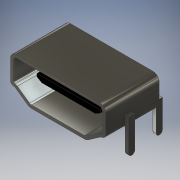
# Autodesk Inventor part: HDMI_Conn
Saved by Autodesk Inventor 2016 (Build 200138000, 138)
## iProperties
Created: 2017-03-02
Part Number: HDMI_Conn
Material: Generic
Document SubType Name: Modeling
Designer: jfixelle
Density: 1 g/cm^3
Appearance: Default
Author: jfixelle
Autodesk Inventor part; units mm, degrees
sketch "Sketch1" plane through (0, 0, 0) normal (0, 0, 1) x (1, 0, 0)
  line L0 (-6.5, 3.1) -> (6.5, 3.1)
  line L1 (7.5, 2.1) -> (7.5, -0.941077)
  line L2 (4.184701, -3.1) -> (-4.184701, -3.1)
  line L3 (-7.5, -0.941077) -> (-7.5, 2.1)
  line L4 (-4.758278, -2.919152) -> (-6.675075, -1.576996)
  line L5 (4.758278, -2.919152) -> (6.675075, -1.576996)
  line L6 (-6.747295, -1.526427) -> (-6.402425, -1.033902)
  line L7 (-6.747295, -1.526427) -> (6.747295, -1.526427)
  line L8 (6.832454, -1.503609) -> (7.12941, -1.42404)
  line L9 (-6.832454, -1.503609) -> (-7.12941, -1.42404)
  arc A0 (-6.675075, -1.576996) -> (-6.832454, -1.503609) centre (-6.961864, -1.986572) ccw
  arc A1 (-7.5, -0.941077) -> (-7.12941, -1.42404) centre (-7, -0.941077) ccw
  arc A2 (6.832454, -1.503609) -> (6.675075, -1.576996) centre (6.961864, -1.986572) ccw
  arc A3 (7.12941, -1.42404) -> (7.5, -0.941077) centre (7, -0.941077) ccw
  arc A4 (-6.5, 3.1) -> (-7.5, 2.1) centre (-6.5, 2.1) ccw
  arc A5 (7.5, 2.1) -> (6.5, 3.1) centre (6.5, 2.1) ccw
  arc A6 (4.184701, -3.1) -> (4.758278, -2.919152) centre (4.184701, -2.1) ccw
  arc A7 (-4.758278, -2.919152) -> (-4.184701, -3.1) centre (-4.184701, -2.1) ccw
  line L10 (-7, 2.1) -> (-7, -0.749246)
  arc A8 (-7, -0.941077) -> (-7, -0.941077) centre (-7, -0.941077) ccw
  line L11 (-6.814705, -0.990727) -> (-6.703044, -1.020646)
  arc A9 (-6.388287, -1.16742) -> (-6.703044, -1.020646) centre (-6.961864, -1.986572) ccw
  line L12 (-6.388287, -1.16742) -> (-4.471489, -2.509576)
  arc A10 (-4.471489, -2.509576) -> (-4.184701, -2.6) centre (-4.184701, -2.1) ccw
  line L13 (-4.184701, -2.6) -> (4.184701, -2.6)
  arc A11 (4.184701, -2.6) -> (4.471489, -2.509576) centre (4.184701, -2.1) ccw
  line L14 (4.471489, -2.509576) -> (6.388287, -1.16742)
  arc A12 (6.703044, -1.020646) -> (6.388287, -1.16742) centre (6.961864, -1.986572) ccw
  line L15 (6.703044, -1.020646) -> (6.814705, -0.990727)
  arc A13 (7, -0.941077) -> (7, -0.941077) centre (7, -0.941077) ccw
  line L16 (7, -0.749246) -> (7, 2.1)
  arc A14 (7, 2.1) -> (6.5, 2.6) centre (6.5, 2.1) ccw
  line L17 (6.5, 2.6) -> (-6.5, 2.6)
  arc A15 (-6.5, 2.6) -> (-7, 2.1) centre (-6.5, 2.1) ccw
  arc A16 (-7, -0.749246) -> (-6.814705, -0.990727) centre (-6.75, -0.749246) ccw
  arc A17 (6.814705, -0.990727) -> (7, -0.749246) centre (6.750001, -0.749246) ccw
  point P0 (0, 0)
  point P1 (-7.5, 3.1)
  point P2 (7.5, -3.1)
  point P3 (7.5, 3.1)
  point P4 (-7.5, -3.1)
  point P5 (-4.5, -3.1)
  point P6 (-7.5, -0.999377)
  point P7 (4.5, -3.1)
  point P8 (7.5, -0.999377)
  dimension "d1" = 15
  dimension "d2" = 7.5
  dimension "d3" = 6.2
  dimension "d4" = 3.1
  dimension "d5" = 9
  dimension "d6" = 4.5
  dimension "d7" = 35
  dimension "d8" = 35
  dimension "d11" = 90
  dimension "d12" = 0.52705
  dimension "d13" = 15
  dimension "d14" = 15
  dimension "d15" = 0.5
  dimension "d16" = 1
  dimension "d17" = 14
  dimension "d18" = 0.25
  constraints: 36 end point, 32 point on circle, 24 point on line, 20 tangent, 18 centre point, 7 equal radius, 4 coincident with centre, 4 parallel, 3 perpendicular, 1 horizontal, 15 other
  measures "d1" distance of point (-7.5, 3.1) point (7.5, 3.1)
  measures "d2" distance from line of point (0, 0) L1
  measures "d3" distance of point (7.5, 3.1) point (7.5, -3.1)
  measures "d4" distance from line of point (0, 0) L0
  measures "d5" distance of point (-4.5, -3.1) point (4.5, -3.1)
  measures "d6" horizontal distance of point (0, 0) point (4.5, -3.1)
  measures "d7" angle of L2 L5
  measures "d8" angle of L2 L4
  measures "d11" angle of L4 L6
  measures "d12" vertical distance of point (-7.5, -0.999) L6.start
  measures "d13" angle of L2 L9
  measures "d14" angle of L2 L8
  measures "d15" radius of A0
  measures "d16" radius of A4
  measures "d17" distance between parallel lines of L10 L16
  measures "d18" radius of A16
sketch "Sketch1 outline for Extrusion1" plane through (0, 0, 0) normal (0, 0, 1) x (1, 0, 0)
  arc A0 (-6.832454, -1.503609) -> (-6.675075, -1.576996) centre (-6.961864, -1.986572) cw
  line L0 (-7.12941, -1.42404) -> (-6.832454, -1.503609)
  line L1 (-6.675075, -1.576996) -> (-4.758278, -2.919152)
  arc A1 (-7.5, -0.941077) -> (-7.12941, -1.42404) centre (-7, -0.941077) ccw
  arc A2 (-4.758278, -2.919152) -> (-4.184701, -3.1) centre (-4.184701, -2.1) ccw
  line L2 (-7.5, 2.1) -> (-7.5, -0.941077)
  line L3 (-4.184701, -3.1) -> (4.184701, -3.1)
  arc A3 (-6.5, 3.1) -> (-7.5, 2.1) centre (-6.5, 2.1) ccw
  arc A4 (4.184701, -3.1) -> (4.758278, -2.919152) centre (4.184701, -2.1) ccw
  line L4 (6.5, 3.1) -> (-6.5, 3.1)
  line L5 (4.758278, -2.919152) -> (6.675075, -1.576996)
  arc A5 (7.5, 2.1) -> (6.5, 3.1) centre (6.5, 2.1) ccw
  arc A6 (6.675075, -1.576996) -> (6.832454, -1.503609) centre (6.961864, -1.986572) cw
  line L6 (7.5, -0.941077) -> (7.5, 2.1)
  line L7 (6.832454, -1.503609) -> (7.12941, -1.42404)
  arc A7 (7.12941, -1.42404) -> (7.5, -0.941077) centre (7, -0.941077) ccw
  arc A8 (-6.5, 2.6) -> (-7, 2.1) centre (-6.5, 2.1) ccw
  line L8 (-7, 2.1) -> (-7, -0.749246)
  arc A9 (-7, -0.749246) -> (-6.814705, -0.990727) centre (-6.75, -0.749246) ccw
  line L9 (-6.814705, -0.990727) -> (-6.703044, -1.020646)
  arc A10 (-6.703044, -1.020646) -> (-6.388287, -1.16742) centre (-6.961864, -1.986572) cw
  line L10 (-6.388287, -1.16742) -> (-4.471489, -2.509576)
  arc A11 (-4.471489, -2.509576) -> (-4.184701, -2.6) centre (-4.184701, -2.1) ccw
  line L11 (-4.184701, -2.6) -> (4.184701, -2.6)
  arc A12 (4.184701, -2.6) -> (4.471489, -2.509576) centre (4.184701, -2.1) ccw
  line L12 (4.471489, -2.509576) -> (6.388287, -1.16742)
  arc A13 (6.388287, -1.16742) -> (6.703044, -1.020646) centre (6.961864, -1.986572) cw
  line L13 (6.703044, -1.020646) -> (6.814705, -0.990727)
  arc A14 (6.814705, -0.990727) -> (7, -0.749246) centre (6.750001, -0.749246) ccw
  line L14 (7, -0.749246) -> (7, 2.1)
  arc A15 (7, 2.1) -> (6.5, 2.6) centre (6.5, 2.1) ccw
  line L15 (6.5, 2.6) -> (-6.5, 2.6)
extrude "Extrusion1" add sketch "Sketch1 outline for Extrusion1" along normal blind 8.47
sketch "Sketch2" plane through (0, 0, 0) normal (0, 0, 1) x (1, 0, 0)
  line L0 (-5, 0.45) -> (5, 0.45)
  line L1 (5, 0.45) -> (5, -0.45)
  line L2 (5, -0.45) -> (-5, -0.45)
  line L3 (-5, -0.45) -> (-5, 0.45)
  line L4 (-5, 0) -> (-4.220577, -0.45)
  line L5 (5, 0) -> (4.220577, -0.45)
  point P0 (0, 0)
  dimension "d21" = 10
  dimension "d22" = 5
  dimension "d23" = 0.9
  dimension "d24" = 0.45
  dimension "d25" = 30
  dimension "d26" = 30
  constraints: 12 end point, 2 midpoint, 2 parallel, 2 point on line, 1 horizontal, 1 perpendicular
  measures "d21" distance of L0.start L0.end
  measures "d22" distance from line of point (0, 0) L1
  measures "d23" distance of L0.end L1.end
  measures "d24" distance from line of point (0, 0) L2
  measures "d25" angle of L2 L4
  measures "d26" angle of L2 L5
extrude "Extrusion2" add sketch "Sketch2" along normal blind 6.8 contours L0 L1 L5 L2 L4 L3
sketch "Sketch3" plane through (0, 0, 0) normal (0, 0, -1) x (-1, 0, 0)
  line L0 (-7.086444, -1.166645) -> (-7.254997, -0.78357)
  line L1 (-7.254997, -0.78357) -> (-7.254997, 2.1)
  line L2 (-7.5, -0.941077) -> (-7.5, 2.1)
  line L3 (-7.254997, 2.1) -> (-6.96386, 2.740724)
  line L4 (-6.96386, 2.740724) -> (-6.560758, 2.918089)
  line L5 (-6.560758, 2.918089) -> (6.612333, 2.918089)
  line L6 (-6.5, 3.1) -> (6.5, 3.1)
  line L7 (6.612333, 2.918089) -> (7.092769, 2.631257)
  line L8 (7.092769, 2.631257) -> (7.353507, 2.038671)
  line L9 (7.353507, 2.038671) -> (7.353507, -0.897314)
  line L10 (7.353507, -0.897314) -> (6.633079, -1.214302)
  line L11 (6.633079, -1.214302) -> (4.545608, -2.822358)
  line L12 (4.545608, -2.822358) -> (-4.031433, -2.970703)
  line L13 (-4.031433, -2.970703) -> (-5.723311, -1.786037)
  line L14 (-4.758278, -2.919152) -> (-6.675075, -1.576996)
  line L15 (-5.723311, -1.786037) -> (-7.086444, -1.166645)
  point P0 (0, 0)
  constraints: 26 end point, 5 parallel, 3 perpendicular
extrude "Extrusion3" add sketch "Sketch3" against normal blind 2
ref_plane "Work Plane1" through (0.25, 0, 0) normal (1, 0, 0) x (0, 1, 0)
sketch "Sketch4" plane through (0.25, 0, 0) normal (1, 0, 0) x (0, 1, 0)
  line L0 (-0.450212, 1.862948) -> (-0.450212, -0.585488)
  line L1 (2.1, 0) -> (-0.941077, 0)
  line L2 (-0.450212, -0.585488) -> (-3.02, -1.038611)
  line L3 (-3.02, -1.038611) -> (-3.02, -1.63)
  line L4 (-3.02, -1.63) -> (-3.1, -1.63)
  line L5 (-3.1, -1.63) -> (-3.1, -0.971383)
  line L6 (-3.1, -0.971383) -> (-0.565386, -0.524462)
  line L7 (-0.565386, -0.524462) -> (-0.565386, 1.862948)
  line L8 (-0.565386, 1.862948) -> (-0.450212, 1.862948)
  line L9 (-3.1, 0) -> (-3.1, 8.47)
  point P0 (0, 0)
  dimension "d32" = 1.63
  dimension "d33" = 0
  dimension "d34" = 0.08
  dimension "d35" = 80
  constraints: 16 end point, 4 perpendicular, 3 parallel
  measures "d32" distance between parallel lines of L4 L1
  measures "d33" distance between parallel lines of L9 L5
  measures "d34" distance of L3.end L4.end
  measures "d35" angle of L3 L2
extrude "Extrusion4" add sketch "Sketch4" along normal mid plane 0.2
pattern_linear "Rectangular Pattern1" count 19 spacing 0.5 along (-1, 0, 0) of "Extrusion4" first direction both ways yes
ref_plane "Work Plane38" through (7.25, 0, 0) normal (1, 0, 0) x (0, 1, 0)
sketch "Sketch5" plane through (7.25, 0, 0) normal (1, 0, 0) x (0, 1, 0)
  line L0 (-5.12, -0.5) -> (-0.210815, -0.5)
  line L1 (-0.210815, -0.5) -> (-0.210815, 0.5)
  line L2 (-0.210815, 0.5) -> (-5.12, 0.5)
  line L3 (-5.12, 0.5) -> (-5.12, -0.5)
  line L4 (-0.941077, 8.47) -> (2.1, 8.47)
  line L5 (-3.1, 0) -> (-3.1, 8.47)
  arc A0 (-4.62, 0.5) -> (-4.62, -0.5) centre (-4.62, 0) ccw
  line L6 (-1.576996, 0) -> (-2.919152, 0)
  point P0 (0, 0)
  dimension "d42" = 1
  dimension "d44" = 2.02
  dimension "d56" = 0.5
  constraints: 8 end point, 3 tangent, 2 parallel, 2 point on circle, 2 point on line, 1 centre point, 1 horizontal, 1 perpendicular
  measures "d42" distance of L2.end L0.start
  measures "d44" distance between parallel lines of L5 L3
  measures "d56" distance between parallel lines of L6 L0
extrude "Extrusion5" add sketch "Sketch5" along normal mid plane 0.5 contours A0 L2 L1 L0
ref_plane "Work Plane39" through (7.85, 0, 0) normal (1, 0, 0) x (0, 1, 0)
sketch "Sketch6" plane through (7.85, 0, 0) normal (1, 0, 0) x (0, 1, 0)
  line L0 (0.317308, 5.45) -> (-5.12, 5.45)
  line L1 (-5.12, 5.45) -> (-5.12, 4.45)
  line L2 (-5.12, 4.45) -> (0.317308, 4.45)
  line L3 (0.317308, 4.45) -> (0.317308, 5.45)
  line L4 (-3.1, 0) -> (-3.1, 8.47)
  arc A0 (-4.62, 5.45) -> (-4.62, 4.45) centre (-4.62, 4.95) ccw
  line L5 (-0.941077, 8.47) -> (2.1, 8.47)
  point P0 (0, 0)
  dimension "d48" = 1
  dimension "d49" = 2.02
  dimension "d55" = 3.02
  constraints: 8 end point, 3 tangent, 2 parallel, 2 point on circle, 2 point on line, 1 centre point, 1 horizontal, 1 perpendicular
  measures "d48" distance of L0.end L1.end
  measures "d49" distance between parallel lines of L1 L4
  measures "d55" distance between parallel lines of L5 L0
extrude "Extrusion6" add sketch "Sketch6" along normal mid plane 0.5 contours L0 L4 L2 A0 | L0 L3 L2 L4
sketch "Sketch7" plane through (7.6, 0, 0) normal (-1, 0, 0) x (0, 0, 1)
  line L0 (4.45, -4.62) -> (4.45, 0.317308)
  line L1 (5.45, 0.317308) -> (5.45, -4.62)
  line L2 (4.45, 0.317308) -> (5.45, 0.317308)
  line L3 (5.45, 0.317308) -> (5.45, -1.198955)
  line L4 (5.45, -1.198955) -> (4.45, -1.198955)
  line L5 (4.45, -1.198955) -> (4.45, 0.317308)
  point P0 (0, 0)
  constraints: 8 end point, 2 parallel, 1 horizontal, 1 perpendicular, 1 point on line
extrude "Extrusion7" add sketch "Sketch7" along normal blind 0.5
mirror "Mirror1" about plane through (0, 0, 0) normal (1, 0, 0) of "Extrusion5", "Extrusion6", "Extrusion7"
ref_plane "Work Plane2" through (-0.5, 0, 0) normal (1, 0, 0) x (0, 1, 0)
ref_plane "Work Plane3" through (0.5, 0, 0) normal (1, 0, 0) x (0, 1, 0)
ref_plane "Work Plane4" through (-1, 0, 0) normal (1, 0, 0) x (0, 1, 0)
ref_plane "Work Plane5" through (1, 0, 0) normal (1, 0, 0) x (0, 1, 0)
ref_plane "Work Plane6" through (-1.5, 0, 0) normal (1, 0, 0) x (0, 1, 0)
ref_plane "Work Plane7" through (1.5, 0, 0) normal (1, 0, 0) x (0, 1, 0)
ref_plane "Work Plane8" through (-2, 0, 0) normal (1, 0, 0) x (0, 1, 0)
ref_plane "Work Plane9" through (2, 0, 0) normal (1, 0, 0) x (0, 1, 0)
ref_plane "Work Plane10" through (-2.5, 0, 0) normal (1, 0, 0) x (0, 1, 0)
ref_plane "Work Plane11" through (2.5, 0, 0) normal (1, 0, 0) x (0, 1, 0)
ref_plane "Work Plane12" through (-3, 0, 0) normal (1, 0, 0) x (0, 1, 0)
ref_plane "Work Plane13" through (3, 0, 0) normal (1, 0, 0) x (0, 1, 0)
ref_plane "Work Plane14" through (-3.5, 0, 0) normal (1, 0, 0) x (0, 1, 0)
ref_plane "Work Plane15" through (3.5, 0, 0) normal (1, 0, 0) x (0, 1, 0)
ref_plane "Work Plane16" through (-4, 0, 0) normal (1, 0, 0) x (0, 1, 0)
ref_plane "Work Plane17" through (4, 0, 0) normal (1, 0, 0) x (0, 1, 0)
ref_plane "Work Plane18" through (-4.5, 0, 0) normal (1, 0, 0) x (0, 1, 0)
ref_plane "Work Plane19" through (4.5, 0, 0) normal (1, 0, 0) x (0, 1, 0)
ref_plane "Work Plane20" through (-0.25, 0, 0) normal (1, 0, 0) x (0, 1, 0)
ref_plane "Work Plane21" through (0.75, 0, 0) normal (1, 0, 0) x (0, 1, 0)
ref_plane "Work Plane22" through (-0.75, 0, 0) normal (1, 0, 0) x (0, 1, 0)
ref_plane "Work Plane23" through (1.25, 0, 0) normal (1, 0, 0) x (0, 1, 0)
ref_plane "Work Plane24" through (-1.25, 0, 0) normal (1, 0, 0) x (0, 1, 0)
ref_plane "Work Plane25" through (1.75, 0, 0) normal (1, 0, 0) x (0, 1, 0)
ref_plane "Work Plane26" through (-1.75, 0, 0) normal (1, 0, 0) x (0, 1, 0)
ref_plane "Work Plane27" through (2.25, 0, 0) normal (1, 0, 0) x (0, 1, 0)
ref_plane "Work Plane28" through (-2.25, 0, 0) normal (1, 0, 0) x (0, 1, 0)
ref_plane "Work Plane29" through (2.75, 0, 0) normal (1, 0, 0) x (0, 1, 0)
ref_plane "Work Plane30" through (-2.75, 0, 0) normal (1, 0, 0) x (0, 1, 0)
ref_plane "Work Plane31" through (3.25, 0, 0) normal (1, 0, 0) x (0, 1, 0)
ref_plane "Work Plane32" through (-3.25, 0, 0) normal (1, 0, 0) x (0, 1, 0)
ref_plane "Work Plane33" through (3.75, 0, 0) normal (1, 0, 0) x (0, 1, 0)
ref_plane "Work Plane34" through (-3.75, 0, 0) normal (1, 0, 0) x (0, 1, 0)
ref_plane "Work Plane35" through (4.25, 0, 0) normal (1, 0, 0) x (0, 1, 0)
ref_plane "Work Plane36" through (-4.25, 0, 0) normal (1, 0, 0) x (0, 1, 0)
ref_plane "Work Plane37" through (4.75, 0, 0) normal (1, 0, 0) x (0, 1, 0)
body "Solid1"
